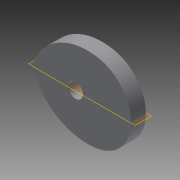
# Autodesk Inventor part: Cam disc Polyline
Saved by Autodesk Inventor 2015 (Build 190141000, 141)
## iProperties
Created: 2008-06-10
Part Number: Cam disc Polyline
Document SubType Name: Modeling
Designer: tangg
Density: 1 g/cm^3
Mass: 6.8214 g
Surface Area: 30.2978 cm^2
Volume: 6.8214 cm^3
Material: Generic
Appearance: Default
Author: tangg
Autodesk Inventor part; units mm, degrees
ref_plane "YZ Plane" through (0, 0, 0) normal (1, 0, 0) x (0, 1, 0)
ref_plane "XY Plane" through (0, 0, 0) normal (0, 0, 1) x (1, 0, 0)
sketch "Sketch6" plane through (0, 0, 0) normal (0, 0, 1) x (1, 0, 0)
  arc A0 (-16.2362, 5.1697) -> (-16.2362, -5.1697) centre (-7.62, 0) ccw
  arc A1 (9.9552, 16.756) -> (-16.2362, 5.1697) centre (5.08, -7.62) ccw
  arc A2 (9.9552, -16.756) -> (9.9552, 16.756) centre (6.604, 0) ccw
  line L0 (-27.0242, 0) -> (35.6389, 0) projected
  arc A3 (-16.2362, 5.1697) -> (-16.2362, -5.1697) centre (-7.62, 0) ccw
  arc A4 (-16.2362, -5.1697) -> (9.9552, -16.756) centre (5.08, 7.62) ccw
  arc A5 (9.9552, -16.756) -> (23.6918, 0) centre (6.604, 0) ccw
  line L1 (0, -29.2695) -> (0, 29.2695) projected
  circle A6 centre (0, 0) radius 3.175
  dimension "d11" = 7.62
  dimension "d12" = 5.08
  dimension "d13" = 6.35
  dimension "d16" = 6.604
  dimension "d17" = 7.62
  constraints: 13 point on circle, 7 centre point, 5 symmetric about line, 4 tangent, 2 point on line, 1 midpoint, 3 other
  measures "d11" distance from line of L0 A4.centre
  measures "d12" distance from line of L1 A4.centre
  measures "d13" diameter of A6
  measures "d16" distance from line of L1 A2.centre
  measures "d17" distance from line of L1 A0.centre
extrude "Extrusion2" add sketch "Sketch6" along normal blind 6.35 contours A1 L1 A6 L0 A0 | L0 A6 L1 A4 A0 | A1 A2 L0 A6 L1 | L1 A6 L0 A2 A4
body "Solid1"
